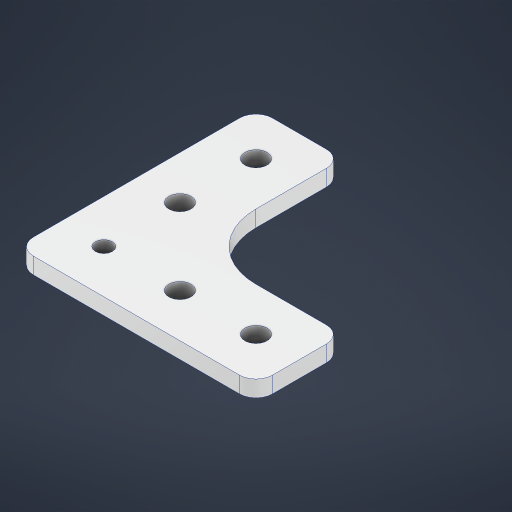
# Autodesk Inventor part: STRU_016_FrameBracket2_90
Saved by Autodesk Inventor 2024.2 (Build 282272000, 272)
## iProperties
Created: 2024-07-25
Part Number: STRU_016_FrameBracket2_90
Material: Aluminum 6061
Document SubType Name: Modeling
Designer: Bryan
Density: 2.7 g/cm^3
Appearance: Aluminum - Flat
Author: Bryan
Autodesk Inventor part; units mm, degrees
ref_plane "YZ Plane" through (0, 0, 0) normal (1, 0, 0) x (0, 1, 0)
ref_plane "XZ Plane" through (0, 0, 0) normal (0, 1, 0) x (-1, 0, 0)
ref_plane "XY Plane" through (0, 0, 0) normal (0, 0, 1) x (1, 0, 0)
sketch "Sketch1" plane through (0, 0, 0) normal (0, 1, 0) x (-1, 0, 0)
  circle A0 centre (0, 0) radius 2.4892
  circle A1 centre (0, -22.225) radius 3.2512
  circle A2 centre (0, -44.45) radius 3.2512
  circle A3 centre (-22.225, 0) radius 3.2512
  circle A4 centre (-44.45, 0) radius 3.2512
  line L0 (12.7, 12.7) -> (-57.15, 12.7)
  line L1 (-57.15, 12.7) -> (-57.15, -12.7)
  line L2 (-57.15, -12.7) -> (-12.7, -12.7)
  line L3 (-12.7, -12.7) -> (-12.7, -57.15)
  line L4 (-12.7, -57.15) -> (12.7, -57.15)
  line L5 (12.7, -57.15) -> (12.7, 12.7)
  dimension "d0" = 4.9784
  dimension "d1" = 6.5024
  dimension "d2" = 22.225
  dimension "d3" = 22.225
  dimension "d4" = 22.225
  dimension "d5" = 22.225
  dimension "d6" = 12.7
  dimension "d7" = 12.7
  dimension "d8" = 12.7
  dimension "d9" = 12.7
  dimension "d10" = 12.7
  dimension "d11" = 12.7
  constraints: 13 end point, 5 centre point, 3 equal radius, 3 horizontal, 3 vertical, 2 horizontal alignment, 2 vertical alignment, 1 coincident
  measures "d0" diameter of A0
  measures "d1" diameter of A1
  measures "d2" distance of A3.centre point (0, 0)
  measures "d3" distance of A4.centre A3.centre
  measures "d4" distance of A1.centre point (0, 0)
  measures "d5" distance of A2.centre A1.centre
  measures "d6" distance from line of A4.centre L1
  measures "d7" distance from line of L4 A2.centre
  measures "d8" distance from line of point (0, 0) L5
  measures "d9" distance from line of point (0, 0) L0
  measures "d10" distance from line of L3 A2.centre
  measures "d11" distance from line of L2 A4.centre
extrude "Extrusion1" add sketch "Sketch1" along normal blind 4.7625
fillet "Fillet1" radius 19.05 1 edges at (12.7, 2.3813, -12.7)
fillet "Fillet2" radius 4.7625 5 edges at (57.15, 2.3813, -12.7) (57.15, 2.3813, 12.7) (12.7, 2.3813, -57.15) (-12.7, 2.3813, -57.15) (-12.7, 2.3813, 12.7)
body "Solid1"
